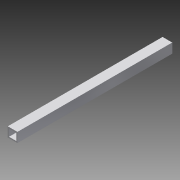
# Autodesk Inventor part: 16inSquarePipe
Saved by Autodesk Inventor 2014 SP2 (Build 180246200, 246)
## iProperties
Created: 2016-04-20
Part Number: 16inSquarePipe
Material: Generic
Document SubType Name: Modeling
Designer: Administrator
Density: 1 g/cm^3
Appearance: Default
Author: Administrator
Autodesk Inventor part; units mm, degrees
ref_plane "YZ Plane" through (0, 0, 0) normal (1, 0, 0) x (0, 1, 0)
ref_plane "XZ Plane" through (0, 0, 0) normal (0, 1, 0) x (-1, 0, 0)
ref_plane "XY Plane" through (0, 0, 0) normal (0, 0, 1) x (1, 0, 0)
sketch "Sketch1" plane through (0, 0, 0) normal (0, 0, 1) x (1, 0, 0)
  line L0 (0, 0) -> (25.4, 0)
  line L1 (25.4, 0) -> (25.4, 25.4)
  line L2 (25.4, 25.4) -> (0, 25.4)
  line L3 (0, 25.4) -> (0, 0)
  line L4 (0, 0) -> (0, 3.175)
  line L5 (0, 3.175) -> (3.175, 3.175)
  line L6 (3.175, 3.175) -> (22.225, 3.175)
  line L7 (22.225, 3.175) -> (22.225, 22.225)
  line L8 (22.225, 22.225) -> (3.175, 22.225)
  line L9 (3.175, 22.225) -> (3.175, 3.175)
  dimension "d0" = 25.4
  dimension "d1" = 25.4
  dimension "d2" = 3.175
  dimension "d3" = 3.175
  dimension "d4" = 19.05
  dimension "d5" = 19.05
  constraints: 20 end point, 4 parallel, 3 perpendicular, 2 horizontal, 1 point on line
  measures "d0" distance of L2.end L1.end
  measures "d1" distance of L1.end L0.end
  measures "d2" distance of L0.start L4.end
  measures "d3" distance of L4.end L5.end
  measures "d4" distance of L8.end L7.end
  measures "d5" distance of L7.end L6.end
extrude "Extrusion1" add sketch "Sketch1" along normal blind 406.4
body "Solid1"
